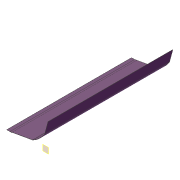
# Autodesk Inventor part: Shovel_Scoop
Saved by Autodesk Inventor 2012 (Build 160160000, 160)
## iProperties
Created: 2013-01-29
Part Number: Shovel_Scoop
Material: Aluminum-6061
Document SubType Name: Modeling
Designer: JesseK
Density: 2.71 g/cm^3
Mass: 398.845 g
Surface Area: 3683.36 cm^2
Volume: 147.175 cm^3
Author: JesseK
Autodesk Inventor part; units mm, degrees
ref_plane "YZ Plane" through (0, 0, 0) normal (1, 0, 0) x (0, 1, 0)
ref_plane "XZ Plane" through (0, 0, 0) normal (0, 1, 0) x (-1, 0, 0)
ref_plane "XY Plane" through (0, 0, 0) normal (0, 0, 1) x (1, 0, 0)
ref_plane "Work Plane1" through (0, 0, 0) normal (0, 0, 1) x (1, 0, 0)
sketch "Sketch1" plane through (0, 0, 0) normal (0, 0, 1) x (1, 0, 0)
  line L0 (-187.1625, 0.7219) -> (-76.4539, 20.4913)
  line L1 (-17.8884, 75.1531) -> (5.459, 162.2869)
  line L2 (5.459, 162.2869) -> (6.2257, 162.0815)
  line L3 (6.2257, 162.0815) -> (-17.1501, 74.8418)
  line L4 (-76.2, 19.7304) -> (-177.8, 1.5875)
  arc A0 (-76.2, 19.7304) -> (-17.1501, 74.8418) centre (-141.0979, 148.4568) ccw
  arc A1 (-76.4539, 20.4913) -> (-17.8884, 75.1531) centre (-141.0979, 148.4568) ccw
  line L5 (-177.8, 1.5875) -> (-177.8, 0)
  line L6 (-177.8, 0) -> (-203.2, 0)
  line L7 (-203.2, 0) -> (-203.2, 0.3587)
  line L8 (-203.2, 0.3587) -> (-187.1625, 0.7219)
  line L9 (0, 0) -> (0, 25.4) construction
  line L10 (0, 25.4) -> (-44.45, 25.4) construction
  line L11 (-44.45, 25.4) -> (-177.8, 1.5875) construction
  line L12 (-177.8, 1.5875) -> (-177.8, 0) construction
  line L13 (-177.8, 0) -> (0, 0) construction
  dimension "d0" = 0.7937
  dimension "d1" = 0.7937
  dimension "d4" = 76.2
  dimension "d8" = 1.5875
  dimension "d9" = 0
  dimension "d11" = 177.8
  dimension "d12" = 25.4
  dimension "d13" = 44.45
  dimension "d14" = 15
  dimension "d15" = 0.7937
  dimension "d16" = 25.4
  constraints: 28 end point, 4 point on circle, 4 vertical, 3 horizontal, 2 centre point, 2 parallel, 1 coincident, 1 collinear, 1 perpendicular
  measures "d0" radial gap between concentric circles of A0 A1
  measures "d1" distance between parallel lines of L0 L4
  measures "d4" horizontal distance of L9.start L4.start
  measures "d8" distance of L4.end L5.end
  measures "d9" vertical distance of L9.start L5.end
  measures "d11" distance of L9.start L5.end
  measures "d12" distance of L5.end L6.end
  measures "d13" horizontal distance of L9.start L10.end
  measures "d14" angle of L9 L3
  measures "d15" distance between parallel lines of L3 L1
  measures "d16" distance between parallel lines of L13 L10
extrude "Extrusion1" add sketch "Sketch1" against normal blind 609.6
body "Solid1"
